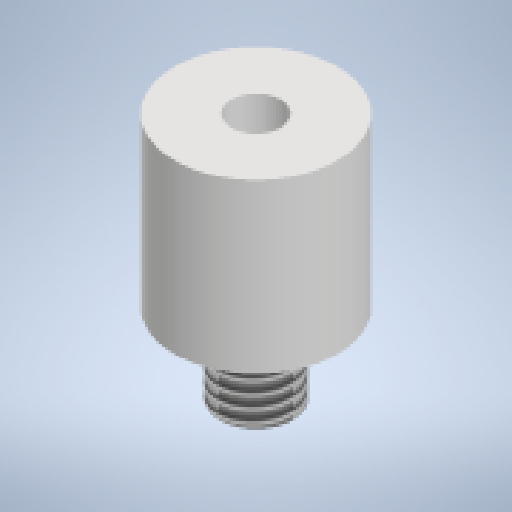
# Autodesk Inventor part: 042
Saved by Autodesk Inventor 2023 (Build 270158000, 158)
## iProperties
Created: 2022-05-02
Part Number: 042
Material: Generic
Document SubType Name: Modeling
Designer: vmiguel
Density: 1 g/cm^3
Appearance: Default
Author: vmiguel
Autodesk Inventor part; units mm, degrees
ref_plane "YZ Plane" through (0, 0, 0) normal (1, 0, 0) x (0, 1, 0)
ref_plane "XZ Plane" through (0, 0, 0) normal (0, 1, 0) x (-1, 0, 0)
ref_plane "XY Plane" through (0, 0, 0) normal (0, 0, 1) x (1, 0, 0)
sketch "Sketch1" plane through (0, 0, 0) normal (1, 0, 0) x (0, 1, 0)
  line L0 (0, -1) -> (-5, -1)
  line L1 (-5, -1) -> (-5, 0)
  line L2 (-4.5, -3.5) -> (-6.8, -3.5)
  line L3 (-6, -1.5) -> (-13, -1.5)
  line L4 (-13, -1.5) -> (-13, 0)
  line L5 (-6, -1.5) -> (-6, -3)
  line L6 (-6, -3) -> (-6.8, -3)
  line L7 (-6.8, -3) -> (-6.8, -3.5)
  line L8 (0, 0) -> (-1.5156, 0)
  line L9 (-5, 0) -> (-13, 0)
  line L10 (0, -1) -> (0, -1.75)
  line L11 (0, -1.75) -> (-4.5, -1.75)
  line L12 (-4.5, -1.75) -> (-4.5, -3.5)
  dimension "d4" = 0.5
  dimension "d5" = 1.5
  dimension "d6" = 0.8
  dimension "d7" = 1
  dimension "d11" = 8
  dimension "d12" = 2
  dimension "d13" = 5
  dimension "d14" = 3
  dimension "d15" = 1.5
  dimension "d16" = 3.5
  dimension "d17" = 7
  constraints: 26 end point, 5 perpendicular, 4 horizontal, 2 vertical, 1 horizontal alignment, 1 vertical alignment
  measures "d4" distance of L6.end L2.end
  measures "d5" distance of L3.start L5.end
  measures "d6" distance of L5.end L6.end
  measures "d7" distance between parallel lines of L1 L5
  measures "d11" distance between parallel lines of L1 L4
  measures "d12" diameter of L0 L8
  measures "d13" distance of L0.start L0.end
  measures "d14" diameter of L3 L8
  measures "d15" distance between parallel lines of L12 L5
  measures "d16" diameter of L11 L8
  measures "d17" diameter of L2 L8
revolve "Revolution1" add sketch "Sketch1" angle 360 about axis through (0, 0, 0) along (0, -1, 0)
thread "Thread1" size "M3x0.5" class "6g" standard "ANSI Metric M Profile" length 5
body "Solid1"
